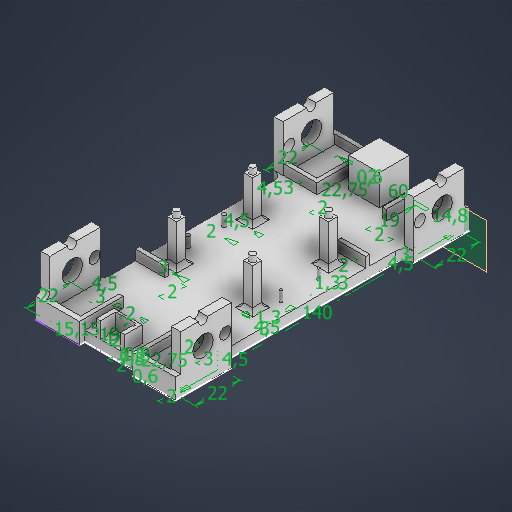
# Autodesk Inventor part: MainBody
Saved by Autodesk Inventor 2026.1 (Build 301233000, 233)
## iProperties
Created: 2026-05-04
Part Number: MainBody
Material: Generic
Document SubType Name: Modeling
Designer: 25adoh
Density: 1 g/cm^3
Appearance: Default
Author: 25adoh
Autodesk Inventor part; units mm, degrees
ref_plane "YZ Plane" through (0, 0, 0) normal (1, 0, 0) x (0, 1, 0)
ref_plane "XZ Plane" through (0, 0, 0) normal (0, 1, 0) x (-1, 0, 0)
ref_plane "XY Plane" through (0, 0, 0) normal (0, 0, 1) x (1, 0, 0)
sketch "Sketch1" plane through (0, 0, 0) normal (0, 1, 0) x (-1, 0, 0)
  line L0 (0, 0) -> (-60, 0)
  line L1 (-60, 0) -> (-60, -140)
  line L2 (-60, -140) -> (0, -140)
  line L3 (0, -140) -> (0, 0)
  line L4 (0, 0) -> (4.5, 0)
  line L5 (4.5, 0) -> (4.5, -22)
  line L6 (4.5, -22) -> (0, -22)
  line L7 (0, -22) -> (0, 0)
  line L8 (-60, 0) -> (-64.5, 0)
  line L9 (-64.5, 0) -> (-64.5, -22)
  line L10 (-64.5, -22) -> (-60, -22)
  line L11 (-60, -22) -> (-60, 0)
  line L12 (0, -140) -> (4.5, -140)
  line L13 (4.5, -140) -> (4.5, -118)
  line L14 (4.5, -118) -> (0, -118)
  line L15 (0, -118) -> (0, -140)
  line L16 (-60, -140) -> (-64.5, -140)
  line L17 (-64.5, -140) -> (-64.5, -118)
  line L18 (-64.5, -118) -> (-60, -118)
  line L19 (-60, -118) -> (-60, -140)
  line L20 (-44.8503, -121.0032) -> (-42.8503, -121.0032)
  line L21 (-42.8503, -121.0032) -> (-42.8503, -140)
  line L22 (-15.15, 0) -> (-15.15, -19)
  line L23 (-15.15, -19) -> (-17.15, -19)
  line L24 (-17.15, -19) -> (-17.15, 0)
  line L25 (-17.15, 0) -> (-15.15, 0)
  line L26 (-16.5, -140) -> (-14.5, -140)
  line L27 (-45.2, -140) -> (-42.8503, -140)
  line L28 (-46, -97.8) -> (-60, -97.8)
  line L29 (-46, -97.8) -> (-46, -95.8)
  line L30 (-46, -95.8) -> (-60, -95.8)
  line L31 (0, 0) -> (-15.15, 0)
  line L32 (-14.5, -42.2) -> (0, -42.2)
  line L33 (-43.5, 0) -> (-43.5, -22.75)
  line L34 (-45.5, 0) -> (-45.5, -22.75)
  line L35 (-45.5, -22.75) -> (-43.5, -22.75)
  line L36 (-43.5, -22.75) -> (-43.5, -24.75)
  line L37 (-43.5, 0) -> (-45.5, 0)
  line L38 (-43.5, -24.75) -> (-60, -24.75)
  line L39 (-45.5, -22.75) -> (-60, -22.75)
  line L40 (-14.5, -140) -> (-14.5, -117.25)
  line L41 (-14.5, -117.25) -> (0, -117.25)
  line L42 (-16.5, -140) -> (-16.5, -117.25)
  line L43 (-16.5, -117.25) -> (-14.5, -117.25)
  line L44 (-16.5, -117.25) -> (-16.5, -115.25)
  line L45 (-16.5, -115.25) -> (0, -115.25)
  line L46 (-45.5, 0) -> (-45.5, 0.6)
  line L47 (-60, 0) -> (-60, 0.6)
  line L48 (-60, 0.6) -> (-45.5, 0.6)
  line L49 (-60, 0.6) -> (-60, 2.6)
  line L50 (-60, 2.6) -> (-43.5, 2.6)
  line L51 (-43.5, 2.6) -> (-43.5, 0)
  line L52 (-16.5, -140) -> (-16.5, -140.6)
  line L53 (-16.5, -140.6) -> (0, -140.6)
  line L54 (-16.5, -140.6) -> (-16.5, -142.6)
  line L55 (-16.5, -142.6) -> (0, -142.6)
  line L56 (0, -142.6) -> (0, -140.6)
  line L57 (0, -140.6) -> (0, -140)
  line L58 (-14.5, -140) -> (-14.5, -140.6)
  line L59 (-25, -140) -> (-25, 0)
  line L60 (-17.15, 0) -> (0, 0)
  line L61 (0, 0) -> (0, 2.6)
  line L62 (0, 2.6) -> (-17.15, 2.6)
  line L63 (-17.15, 2.6) -> (-17.15, 0)
  line L64 (-42.8503, -140) -> (-60, -140)
  line L65 (-60, -140) -> (-60, -142.6)
  line L66 (-60, -142.6) -> (-42.8503, -142.6)
  line L67 (-42.8503, -142.6) -> (-42.8503, -140)
  line L68 (-44.8503, -121.0032) -> (-44.8503, -140)
  circle A0 centre (-11.25, -51.25) radius 1.5
  circle A1 centre (-11.25, -51.25) radius 2.25
  line L69 (-9, -53.5) -> (-13.5, -53.5)
  line L70 (-13.5, -53.5) -> (-13.5, -49)
  line L71 (-13.5, -49) -> (-9, -49)
  line L72 (-9, -49) -> (-9, -53.5)
  circle A2 centre (-48.75, -51.25) radius 1.5
  circle A3 centre (-48.75, -51.25) radius 2.25
  line L73 (-51, -53.5) -> (-46.5, -53.5)
  line L74 (-46.5, -53.5) -> (-46.5, -49)
  line L75 (-46.5, -49) -> (-51, -49)
  line L76 (-51, -49) -> (-51, -53.5)
  circle A4 centre (-48.75, -88.75) radius 1.5
  circle A5 centre (-48.75, -88.75) radius 2.25
  line L77 (-46.5, -86.5) -> (-51, -86.5)
  line L78 (-51, -86.5) -> (-51, -91)
  line L79 (-51, -91) -> (-46.5, -91)
  line L80 (-46.5, -91) -> (-46.5, -86.5)
  circle A6 centre (-11.25, -88.75) radius 1.5
  circle A7 centre (-11.25, -88.75) radius 2.25
  line L81 (-13.5, -86.5) -> (-9, -86.5)
  line L82 (-9, -86.5) -> (-9, -91)
  line L83 (-9, -91) -> (-13.5, -91)
  line L84 (-13.5, -91) -> (-13.5, -86.5)
  line L85 (-14.5, -42.2) -> (-14.5, -44.2)
  line L86 (-14.5, -44.2) -> (0, -44.2)
  circle A8 centre (-7, -79) radius 1
  circle A9 centre (-7, -61) radius 1
  circle A10 centre (-53.3, -60.7) radius 0.65
  circle A11 centre (-53.3, -79.3) radius 0.65
  line L87 (-35, -140) -> (-35, 0)
  line L88 (-64.5, -22) -> (-60, -22)
  line L89 (-60, -22) -> (-60, -25)
  line L90 (-60, -25) -> (-64.5, -25)
  line L91 (-64.5, -25) -> (-64.5, -22)
  line L92 (-64.5, -118) -> (-60, -118)
  line L93 (-60, -118) -> (-60, -115)
  line L94 (-60, -115) -> (-64.5, -115)
  line L95 (-64.5, -115) -> (-64.5, -118)
  line L96 (4.5, -22) -> (0, -22)
  line L97 (0, -22) -> (0, -25)
  line L98 (0, -25) -> (4.5, -25)
  line L99 (4.5, -25) -> (4.5, -22)
  line L100 (4.5, -118) -> (0, -118)
  line L101 (0, -118) -> (0, -115)
  line L102 (0, -115) -> (4.5, -115)
  line L103 (4.5, -115) -> (4.5, -118)
  line L104 (-64.5, 0) -> (-60, 0)
  line L105 (-60, 0) -> (-60, 2.6)
  line L106 (-60, 2.6) -> (-64.5, 2.6)
  line L107 (-64.5, 2.6) -> (-64.5, 0)
  line L108 (0, 2.6) -> (4.5, 2.6)
  line L109 (4.5, 2.6) -> (4.5, 0)
  line L110 (4.5, 0) -> (0, 0)
  line L111 (0, 0) -> (0, 2.6)
  line L112 (0, -142.6) -> (4.5, -142.6)
  line L113 (4.5, -142.6) -> (4.5, -140)
  line L114 (4.5, -140) -> (0, -140)
  line L115 (0, -140) -> (0, -142.6)
  line L116 (-64.5, -140) -> (-60, -140)
  line L117 (-60, -140) -> (-60, -142.6)
  line L118 (-60, -142.6) -> (-64.5, -142.6)
  line L119 (-64.5, -142.6) -> (-64.5, -140)
  line L120 (-25, 0) -> (-35, 0)
  line L121 (-35, 0) -> (-35, -7.5)
  line L122 (-35, -7.5) -> (-25, -7.5)
  line L123 (-25, -7.5) -> (-25, 0)
  line L124 (-35, -7.5) -> (-35, -6.7)
  line L125 (-35, -5.7) -> (-35, -6.7)
  line L126 (-25, 0) -> (-23, 0)
  line L127 (-23, 0) -> (-23, -8)
  line L128 (-23, -8) -> (-25, -8)
  line L129 (-25, -8) -> (-25, 0)
  line L130 (-35, -7.5) -> (-37, -7.5)
  line L131 (-37, -7.5) -> (-37, 0)
  line L132 (-37, 0) -> (-35, 0)
  line L133 (-35, 0) -> (-35, -7.5)
  line L134 (-35, -6.7) -> (-35.3, -6.7)
  line L135 (-35, -6.5) -> (-35, -6.7)
  line L136 (-37, -7.5) -> (-23, -7.5)
  line L137 (-23, -7.5) -> (-23, -8.5)
  line L138 (-23, -8.5) -> (-37, -8.5)
  line L139 (-37, -8.5) -> (-37, -7.5)
  line L140 (-35, -6.7) -> (-35.5, -6.7)
  line L141 (-35.5, -6.7) -> (-35.5, -5.7)
  line L142 (-35.5, -5.7) -> (-35, -5.7)
  line L143 (-35, -5.7) -> (-35, -6.7)
  line L144 (-15.15, 0) -> (0, 0)
  point P0 (-60, -118)
  point P1 (0, -118)
  point P2 (-30, -70)
  point P3 (0, -49.2)
  point P4 (-35, -130)
  point P5 (-12.75, -52.75)
  point P6 (-30, -91.25)
  point P7 (-13.5, -88.75)
  point P8 (-11.25, -91)
  point P9 (-11.25, -86.5)
  point P10 (-9, -88.75)
  point P11 (-9, -51.25)
  point P12 (-11.25, -49)
  point P13 (-11.25, -53.5)
  point P14 (-13.5, -51.25)
  point P15 (-51, -51.25)
  point P16 (-48.75, -49)
  point P17 (-48.75, -53.5)
  point P18 (-46.5, -51.25)
  point P19 (-46.5, -88.75)
  point P20 (-48.75, -91)
  point P21 (-48.75, -86.5)
  point P22 (-51, -88.75)
  dimension "d0" = 60
  dimension "d1" = 140
  dimension "d2" = 4.5
  dimension "d3" = 22
  dimension "d4" = 4.5
  dimension "d5" = 22
  dimension "d6" = 4.5
  dimension "d7" = 22
  dimension "d8" = 4.5
  dimension "d9" = 22
  dimension "d64" = 14.8
  dimension "d66" = 19
  dimension "d67" = 2
  dimension "d74" = 19
  dimension "d75" = 2
  dimension "d100" = 2
  dimension "d107" = 22.75
  dimension "d108" = 2
  dimension "d109" = 22.75
  dimension "d110" = 2
  dimension "d111" = 0.6
  dimension "d112" = 2
  dimension "d113" = 0.6
  dimension "d114" = 2
  dimension "d134" = 3
  dimension "d137" = 3
  dimension "d138" = 4.5
  dimension "d140" = 3
  dimension "d143" = 4.5
  dimension "d148" = 2
  dimension "d154" = 2
  dimension "d160" = 1.3
  dimension "d163" = 1.3
  dimension "d165" = 3
  dimension "d166" = 3
  dimension "d167" = 3
  dimension "d168" = 3
  dimension "d175" = 7.5
  dimension "d176" = 0.8
  dimension "d179" = 2
  dimension "d180" = 2
  dimension "d182" = 1
  dimension "d183" = 0.5
  dimension "d186" = 15.15
  constraints: 286 end point, 48 parallel, 40 perpendicular, 34 horizontal, 17 point on line, 15 vertical, 12 centre point, 4 coincident, 2 collinear, 20 other
  measures "d0" distance of L2.end L1.end
  measures "d1" distance of L1.end L1.start
  measures "d2" distance of L5.end L6.end
  measures "d3" distance of L4.end L5.end
  measures "d4" distance of L10.end L9.end
  measures "d5" distance of L9.end L8.end
  measures "d6" distance of L14.end L13.end
  measures "d7" distance of L13.end L12.end
  measures "d8" distance of L17.end L18.end
  measures "d9" distance of L16.end L17.end
  measures "d64" distance of L1.end L27.start
  measures "d66" distance of L27.start L20.start
  measures "d67" distance of L20.start L20.end
  measures "d74" distance of L22.start L22.end
  measures "d75" distance of L22.end L23.end
  measures "d100" distance of L28.start L29.end
  measures "d107" distance of L33.start L33.end
  measures "d108" distance of L33.end L36.end
  measures "d109" distance of L26.end L40.end
  measures "d110" distance of L42.end L44.end
  measures "d111" distance of L34.start L46.end
  measures "d112" distance of L47.end L49.end
  measures "d113" distance of L26.start L52.end
  measures "d114" distance of L52.end L54.end
  measures "d134" diameter of A0
  measures "d137" diameter of A2
  measures "d138" diameter of A3
  measures "d140" diameter of A4
  measures "d143" diameter of A7
  measures "d148" distance of L32.start L85.end
  measures "d154" diameter of A8
  measures "d160" diameter of A10
  measures "d163" diameter of A11
  measures "d165" distance of L88.end L89.end
  measures "d166" distance of L93.end L92.end
  measures "d167" distance of L97.end L96.end
  measures "d168" distance of L100.end L101.end
  measures "d175" distance of L121.end L120.end
  measures "d176" distance of L121.end L124.end
  measures "d179" distance of L127.end L128.end
  measures "d180" distance of L131.end L132.end
  measures "d182" distance of L136.end L137.end
  measures "d183" distance of L141.end L142.end
  measures "d186" distance of L4.start L22.start
extrude "Extrusion1" add sketch "Sketch1" along normal blind 5 contours L3 L32 L85 L86 L45 L44 L42 L2 L59 L138 L137 L127 L0 L24 L23 L22 | L22 L23 L24 L0 | L127 L136 L59 L0 | L3 L86 L85 L32 | L59 L122 L87 L0 | L127 L128 L59 L136 | L87 L142 L141 L140 L134 L130 L131 L0 | L59 L138 L87 L122 | L137 L138 L59 L128 | L131 L139 L138 L87 L2 L21 L20 L68 L1 L28 L29 L30 L38 L36 L33 L0 | L87 L134 L140 L141 L142 | L87 L138 L139 L130 | L3 L41 L43 L44 L45 | L33 L35 L34 L0 | L0 L46 L48 L49 L50 L51 | L59 L2 L87 L138 | L3 L2 L40 L41 | L34 L39 L1 L0 | L0 L47 L48 L46 | L36 L38 L1 L39 L35 | L40 L2 L42 L43 | L2 L58 L53 L52 | L2 L68 L20 L21 | L57 L53 L58 L2 | L53 L56 L55 L54 | L30 L29 L28 L1 | A0 | A1 | L72 L69 A1 | A1 L71 L72 | A1 L70 L71 | L69 L70 A1 | A2 | A3 | L74 L73 A3 | A3 L75 L74 | A3 L76 L75 | L73 L76 A3 | A4 | A5 | L80 L79 A5 | A5 L77 L80 | A5 L78 L77 | L79 L78 A5 | A6 | A7 | L82 L83 A7 | A7 L81 L82 | A7 L84 L81 | L83 L84 A7 | A8 | A9 | A10 | A11
extrude "Extrusion2" add sketch "Sketch1" along normal blind 28 contours L4 L5 L6 L3 | L6 L99 L98 L3 | L102 L103 L14 L3 | L13 L12 L3 L14 | L1 L10 L9 L8 | L1 L90 L91 L10 | L16 L17 L18 L1 | L18 L95 L94 L1
sketch "Sketch2" plane through (64.5, 0, 0) normal (1, 0, 0) x (0, 0, -1)
  line L0 (0, 28) -> (25, 28) projected
  line L1 (22, 0) -> (22, 28) projected
  line L2 (0, 28) -> (0, 5)
  line L3 (0, 5) -> (22, 5)
  line L4 (0, 28) -> (22, 5)
  line L5 (22, 0) -> (22, 28) projected
  line L6 (0, 5) -> (22, 28)
  circle A0 centre (11, 16.5) radius 5
  line L7 (118, 28) -> (140, 28)
  line L8 (118, 0) -> (118, 28)
  line L9 (140, 0) -> (140, 28)
  line L10 (118, 28) -> (118, 5)
  line L11 (118, 5) -> (140, 5)
  line L12 (118, 28) -> (140, 5)
  line L13 (140, 0) -> (140, 28)
  line L14 (118, 5) -> (140, 28)
  circle A1 centre (129, 16.5) radius 5
  line L15 (118, 28) -> (140, 28) projected
  line L16 (118, 0) -> (118, 28) projected
  line L17 (140, 0) -> (140, 28) projected
  line L18 (0, 28) -> (0, 5)
  line L19 (12.5, 28) -> (11.25, 28) construction
  circle A2 centre (11, 27.75) radius 2.25
  circle A3 centre (129, 27.75) radius 2.25
  circle A4 centre (22, 16.5) radius 2.75
  circle A5 centre (118, 16.5) radius 2.75
  dimension "d14" = 23
  dimension "d15" = 10
  dimension "d16" = 23
  dimension "d17" = 10
  dimension "d60" = 4.5
  dimension "d61" = 4.5
  dimension "d115" = 5.5
  dimension "d116" = 5.5
  constraints: 28 end point, 6 centre point, 5 point on line, 3 midpoint, 3 perpendicular, 2 coincident, 1 horizontal
  measures "d14" distance of L0.start L2.end
  measures "d15" diameter of A0
  measures "d16" distance of L7.start L10.end
  measures "d17" diameter of A1
  measures "d60" diameter of A2
  measures "d61" diameter of A3
  measures "d115" diameter of A4
  measures "d116" diameter of A5
extrude "Extrusion3" cut sketch "Sketch2" against normal up to surface (69 mm away) contours A2 L0 | L0 A2 | A0 L6 L4 | L4 L6 A0 | L6 L4 A0 | L6 A0 L4 | A4 L1 | L1 A4 | A3 L7 | L7 A3 | A5 L8 | L8 A5 | A1 L14 L12 | L12 L14 A1 | L14 A1 L12 | L12 A1 L14
sketch "Sketch4" plane through (0, 5, 0) normal (0, 1, 0) x (1, 0, 0)
  line L0 (60, 140) -> (16.5, 140) projected
  line L1 (17, 140) -> (0, 140) projected
  line L2 (0, 140) -> (-4.5, 140) projected
  line L3 (34, 140) -> (26, 140)
  line L4 (37.5, 140) -> (22.5, 140)
  line L5 (37.5, 140) -> (22.5, 140)
  line L6 (22.5, 140) -> (22.5, 125)
  line L7 (22.5, 125) -> (37.5, 125)
  line L8 (37.5, 125) -> (37.5, 140)
  line L9 (34, 140) -> (26, 140)
  line L10 (26, 140) -> (26, 134)
  line L11 (26, 134) -> (34, 134)
  line L12 (34, 134) -> (34, 140)
  point P0 (0, 0)
  point P1 (30, 140)
  point P2 (30, 140)
  dimension "d32" = 8
  dimension "d33" = 15
  dimension "d34" = 15
  dimension "d35" = 15
  dimension "d36" = 8
  dimension "d37" = 6
  constraints: 20 end point, 4 parallel, 2 horizontal, 2 midpoint, 2 perpendicular, 1 point on line
  measures "d32" distance of L3.start L3.end
  measures "d33" distance of L4.start L4.end
  measures "d34" distance of L7.end L6.end
  measures "d35" distance of L6.end L5.end
  measures "d36" distance of L11.end L10.end
  measures "d37" distance of L10.end L9.end
extrude "Extrusion5" add sketch "Sketch4" along normal blind 15
ref_plane "Work Plane1" through (64.5, 0, -140) normal (0, 0, -1) x (-1, 0, 0)
sketch "Sketch5" plane through (64.5, 0, -140) normal (0, 0, -1) x (-1, 0, 0)
  line L0 (42, 5) -> (42, 20) projected
  line L1 (42, 5) -> (48, 5) projected
  line L2 (4.5, 5) -> (4.5, 28) projected
  line L3 (0, 28) -> (4.5, 28) projected
  line L4 (0, 0) -> (0, 28) projected
  line L5 (34.5, 20) -> (34.5, 5)
  line L6 (27, 5) -> (42, 5) projected
  line L7 (34.5, 5) -> (34.5, 13)
  line L8 (30.5, 13) -> (38.5, 13)
  line L9 (38.5, 13) -> (38.5, 5)
  line L10 (30.5, 13) -> (30.5, 5)
  line L11 (0, 0) -> (48, 0) projected
  line L12 (48, 0) -> (48, 5) projected
  line L13 (42, 5) -> (42, 20) projected
  line L14 (27, 20) -> (42, 20) projected
  line L15 (27, 5) -> (27, 20) projected
  line L16 (4.5, 5) -> (27, 5) projected
  point P0 (64.5, 0)
  point P1 (42, 5)
  dimension "d40" = 8
  dimension "d41" = 8
  constraints: 10 end point, 3 point on line, 2 midpoint, 2 perpendicular, 1 horizontal
  measures "d40" distance of L5.end L7.end
  measures "d41" distance of L8.start L8.end
extrude "Extrusion6" cut sketch "Sketch5" against normal blind 6 contours L6 L5 L8 L9 | L6 L10 L8 L5
extrude "Extrusion7" add sketch "Sketch1" along normal blind 10 contours L61 L108 L109 L4 | L0 L63 L62 L61 | L22 L23 L24 L0 | L3 L86 L85 L32 | L3 L41 L43 L44 L45 | L33 L35 L34 L0 | L0 L46 L48 L49 L50 L51 | L36 L38 L1 L39 L35 | L40 L2 L42 L43 | L113 L112 L56 L57 L12 | L8 L107 L106 L49 L47 | L2 L58 L53 L52 | L67 L66 L65 L2 | L2 L68 L20 L21 | L53 L56 L55 L54 | L118 L119 L16 L65 | L30 L29 L28 L1 | A8 | A9 | A10 | A11
extrude "Extrusion8" add sketch "Sketch1" along normal blind 25 contours A0 | A1 | L72 L69 A1 | A1 L71 L72 | A1 L70 L71 | L69 L70 A1 | A2 | A3 | L74 L73 A3 | A3 L75 L74 | A3 L76 L75 | L73 L76 A3 | A4 | A5 | L80 L79 A5 | A5 L77 L80 | A5 L78 L77 | L79 L78 A5 | A6 | A7 | L82 L83 A7 | A7 L81 L82 | A7 L84 L81 | L83 L84 A7
extrude "Extrusion9" add sketch "Sketch1" along normal blind 28 contours A0 | A2 | A4 | A6
fillet "Fillet1" radius 2 16 edges at (48.75, 5, -49) (46.5, 5, -51.25) (48.75, 5, -53.5) (51, 5, -51.25) (46.5, 5, -88.75) (48.75, 5, -91) (48.75, 5, -86.5) (51, 5, -88.75) (11.25, 5, -86.5) (9, 5, -88.75) (11.25, 5, -91) (13.5, 5, -88.75) (9, 5, -51.25) (11.25, 5, -49) (11.25, 5, -53.5) (13.5, 5, -51.25)
fillet "Fillet2" radius 2.6 2 edges at (62.25, 10, -140) (-2.25, 10, 0)
fillet "Fillet3" radius 4.5 4 edges at (0, 2.5, -25) (0, 2.5, -115) (60, 2.5, -115) (60, 2.5, -25)
extrude "Extrusion12" add sketch "Sketch1" along normal blind 5.5 contours L3 L2 L40 L41 | L34 L39 L1 L0 | L0 L47 L48 L46 | L57 L53 L58 L2 | L53 L56 L55 L54
extrude "Extrusion13" add sketch "Sketch1" along normal blind 13 contours L127 L136 L59 L0 | L127 L128 L59 L136 | L87 L142 L141 L140 L134 L130 L131 L0 | L59 L138 L87 L122 | L137 L138 L59 L128 | L87 L138 L139 L130
body "Solid1"
